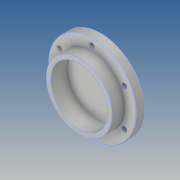
# Autodesk Inventor part: 200-10-ROCKER-BEARING-02
Saved by Autodesk Inventor 2018.2 (Build 222227000, 227)
## iProperties
Manager: feesmrt
Company: FRANCOR
Created: 2017-10-26
Part Number: 200-10-ROCKER-BEARING-02
Material: Aluminium 6061
Document SubType Name: Modeling
Designer: feesmrt
Density: 2.7 g/cm^3
Appearance: Aluminium - flach
Project: Rescue Robot
Cost Center: -
Description: Rocker Bearing Housing Cap
Engineer: feesmrt
Authority: feesmrt
Stock Number: 200-10-ROCKER-BEARING-02
Mass: 208.743 g
Surface Area: 272.937 cm^2
Volume: 77.3121 cm^3
Author: feesmrt
Title: Rocker Bearing Housing Cap
Subject: Rescue Robot
Revision Number: 1
Autodesk Inventor part; units mm, degrees
ref_plane "YZ Plane" through (0, 0, 0) normal (1, 0, 0) x (0, 1, 0)
ref_plane "XZ Plane" through (0, 0, 0) normal (0, 1, 0) x (-1, 0, 0)
ref_plane "XY Plane" through (0, 0, 0) normal (0, 0, 1) x (1, 0, 0)
derived "200-10-ROCKER-BEARING-01.ipt"
sketch "Skizze_Lagersitz" plane through (0, 0, 0) normal (1, 0, 0) x (0, 1, 0)
  line L0 (-12.5, 36) -> (17.5, 36)
  line L1 (-12.5, -36) -> (-12.5, 36)
  line L2 (-17.5, 32.25) -> (-12.5, 32.25)
  line L3 (-17.5, -32.25) -> (-17.5, 32.25)
  line L4 (-32.5, 18) -> (-17.5, 18)
  line L5 (-32.5, -18) -> (-17.5, -18)
  line L6 (-17.5, -32.25) -> (-12.5, -32.25)
  line L7 (-12.5, -36) -> (17.5, -36)
  line L8 (32.5, 36) -> (32.5, -36)
  line L9 (32.5, 50) -> (32.5, -50)
  line L10 (30, -50) -> (30, 0)
  line L11 (-32.5, -18) -> (-32.5, 18)
  line L12 (-32.5, 50) -> (-32.5, -50)
  line L13 (-32.5, -50) -> (-32.5, 50)
  line L14 (-12.5, -36) -> (-12.5, 36)
  line L15 (17.5, -37.5) -> (17.5, 37.5)
  line L16 (17.5, 37.5) -> (32.5, 37.5)
  point P0 (0, 0)
  point P1 (30, 86)
  point P2 (30, 14)
  point P3 (-30, 32)
  point P4 (-30, 68)
sketch "Skizze4" plane through (0, 0, 0) normal (1, 0, 0) x (0, 1, 0)
  line L0 (32.5, 50) -> (42.7, 50)
  line L1 (32.5, 37.5) -> (17.7, 37.5)
  line L2 (17.7, 37.5) -> (17.7, 32.25)
  line L3 (17.7, 32.25) -> (37.7, 32.25)
  line L4 (32.5, 37.5) -> (32.5, 50)
  line L5 (42.7, 50) -> (42.7, 0)
  line L6 (42.7, 0) -> (37.7, 0)
  line L7 (37.7, 0) -> (37.7, 32.25)
  line L8 (17.5, 37.5) -> (32.5, 37.5) construction
  line L9 (-12.5, -36) -> (-12.5, 36) construction
  line L10 (-17.5, 32.25) -> (-12.5, 32.25) construction
  line L11 (0, 113.2) -> (0, -77.2) construction
  line L12 (-47.54, 0) -> (57.74, 0) projected
  point P0 (-15, 32.25)
  dimension "d74" = 5
  dimension "d79" = 30.2
  dimension "d81" = 25
  constraints: 16 end point, 4 perpendicular, 2 horizontal, 1 collinear, 1 horizontal alignment, 1 midpoint
  measures "d74" distance between parallel lines of L5 L7
  measures "d79" distance between parallel lines of L2 L9
  measures "d81" distance between parallel lines of L2 L5
revolve "Grundkoerper" add sketch "Skizze4" angle 360 about axis through (0, 0, 0) along (0, 1, 0)
sketch "Skizze6" plane through (0, 42.7, 0) normal (0, 1, 0) x (1, 0, 0)
  circle A0 centre (0, 0) radius 36 construction
  circle A1 centre (0, 0) radius 50 construction
  circle A2 centre (0, 0) radius 42.5 construction
  line L0 (0, 77.2) -> (0, -113.2) construction
  line L1 (70, 0) -> (-70, 0) construction
  point P0 (0, -42.5)
  point P1 (36.8061, -21.25)
  point P2 (36.8061, 21.25)
  point P3 (0, 42.5)
  point P4 (-36.8061, 21.25)
  point P5 (-36.8061, -21.25)
  dimension "d59" = 85
  dimension "d62" = 360
  constraints: 1 coincident, 1 point on line, 1 vertical alignment, 9 other
hole "DIN7984_M5" at (0, 42.7, 42.5) at (36.8061, 42.7, 21.25) at (36.8061, 42.7, -21.25) at (0, 42.7, -42.5) at (-36.8061, 42.7, -21.25) at (-36.8061, 42.7, 21.25) direction (0, -1, 0) diameter 5.5 end through all counterbore diameter 10 counterbore depth 3.9
chamfer "Fase_Passung" distance 0.3 angle 45 2 edges at (0, 17.7, -32.25) (0, 17.7, -37.5)
chamfer "Fase_Allgemein" distance 0.5 angle 45 2 edges at (0, 32.5, -50) (0, 42.7, -50)
